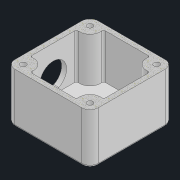
# Autodesk Inventor part: box
Saved by Autodesk Inventor 2021 (Build 250183000, 183)
## iProperties
Created: 2021-04-30
Part Number: box
Material: 一般
Document SubType Name: Modeling
Designer: yuta0
Density: 1 g/cm^3
Appearance: 既定
Author: yuta0
Autodesk Inventor part; units mm, degrees
ref_plane "YZ Plane" through (0, 0, 0) normal (1, 0, 0) x (0, 1, 0)
ref_plane "XZ Plane" through (0, 0, 0) normal (0, 1, 0) x (-1, 0, 0)
ref_plane "XY Plane" through (0, 0, 0) normal (0, 0, 1) x (1, 0, 0)
sketch "スケッチ1" plane through (0, 0, 0) normal (0, 1, 0) x (-1, 0, 0)
  line L0 (25, 25) -> (-25, 25)
  line L1 (-25, 25) -> (-25, -25)
  line L2 (-25, -25) -> (25, -25)
  line L3 (25, -25) -> (25, 25)
  line L4 (25, 25) -> (-25, -25) construction
  line L5 (-25, 25) -> (25, -25) construction
  point P0 (0, 0)
  dimension "d0" = 50
  dimension "d1" = 50
  constraints: 12 end point, 2 midpoint, 2 parallel, 1 horizontal, 1 perpendicular
  measures "d0" distance of L2.end L1.end
  measures "d1" distance of L1.end L0.end
extrude "押し出し1" add sketch "スケッチ1" against normal mid plane 33
fillet "フィレット1" radius 5 4 edges at (25, 0, 25) (25, 0, -25) (-25, 0, 25) (-25, 0, -25)
fillet "フィレット2" radius 1 16 edges at (25, -16.5, 0) (23.5355, -16.5, 23.5355) (0, -16.5, 25) (-23.5355, -16.5, 23.5355) (-25, -16.5, 0) (-23.5355, -16.5, -23.5355) (0, -16.5, -25) (23.5355, -16.5, -23.5355) (23.5355, 16.5, 23.5355) (25, 16.5, 0) (23.5355, 16.5, -23.5355) (0, 16.5, -25) (-23.5355, 16.5, -23.5355) (-25, 16.5, 0) (-23.5355, 16.5, 23.5355) (0, 16.5, 25)
sketch "スケッチ2" plane through (0, 16.5, 0) normal (0, 1, 0) x (1, 0, 0)
  arc A0 (-25, -20) -> (-20, -25) centre (-20, -20) ccw projected
  arc A1 (-20, 25) -> (-25, 20) centre (-20, 20) ccw projected
  arc A2 (25, 20) -> (20, 25) centre (20, 20) ccw projected
  arc A3 (20, -25) -> (25, -20) centre (20, -20) ccw projected
  point P0 (0, 0)
hole "穴1" at (-20, 16.5, -20) at (20, 16.5, 20) at (-20, 16.5, 20) at (20, 16.5, -20) direction (0, -1, 0) diameter 3.4 end through all counterbore diameter 6.5 counterbore depth 3 clearance for "Socket Head Cap Screw" size "M3" standard "Ansi Metric M Profile"
shell "シェル1" thickness 3 removed faces 0
sketch "スケッチ3" plane through (0, -16.5, 0) normal (0, -1, 0) x (1, 0, 0)
  circle A0 centre (20, 20) radius 1.7 projected
  circle A1 centre (-20, 20) radius 1.7 projected
  circle A2 centre (-20, -20) radius 1.7 projected
  line L0 (21.5877, 17.25) -> (18.4123, 17.25)
  line L1 (18.4123, 17.25) -> (16.8246, 20)
  line L2 (16.8246, 20) -> (18.4123, 22.75)
  line L3 (18.4123, 22.75) -> (21.5877, 22.75)
  line L4 (21.5877, 22.75) -> (23.1754, 20)
  line L5 (23.1754, 20) -> (21.5877, 17.25)
  line L6 (-20, 24) -> (20, 24) projected
  circle A3 centre (20, -20) radius 1.7 projected
  line L7 (21.5877, -17.25) -> (23.1754, -20)
  line L8 (23.1754, -20) -> (21.5877, -22.75)
  line L9 (21.5877, -22.75) -> (18.4123, -22.75)
  line L10 (18.4123, -22.75) -> (16.8246, -20)
  line L11 (16.8246, -20) -> (18.4123, -17.25)
  line L12 (18.4123, -17.25) -> (21.5877, -17.25)
  line L13 (-18.4123, -22.75) -> (-21.5877, -22.75)
  line L14 (-21.5877, -22.75) -> (-23.1754, -20)
  line L15 (-23.1754, -20) -> (-21.5877, -17.25)
  line L16 (-21.5877, -17.25) -> (-18.4123, -17.25)
  line L17 (-18.4123, -17.25) -> (-16.8246, -20)
  line L18 (-16.8246, -20) -> (-18.4123, -22.75)
  line L19 (-21.5877, 22.75) -> (-18.4123, 22.75)
  line L20 (-18.4123, 22.75) -> (-16.8246, 20)
  line L21 (-16.8246, 20) -> (-18.4123, 17.25)
  line L22 (-18.4123, 17.25) -> (-21.5877, 17.25)
  line L23 (-21.5877, 17.25) -> (-23.1754, 20)
  line L24 (-23.1754, 20) -> (-21.5877, 22.75)
  point P0 (0, 0)
  dimension "d14" = 5.5
  dimension "d15" = 5.5
  dimension "d16" = 5.5
  dimension "d17" = 5.5
  constraints: 48 end point, 4 coincident, 4 parallel, 52 other
  measures "d14" distance between parallel lines of L3 L0
  measures "d15" distance between parallel lines of L22 L19
  measures "d16" distance between parallel lines of L13 L16
  measures "d17" distance between parallel lines of L9 L12
extrude "押し出し2" cut sketch "スケッチ3" against normal blind 3 contours A0 | A1 | A2 | L0 L1 L2 L3 L4 L5 | A3 | L7 L8 L9 L10 L11 L12 | L13 L14 L15 L16 L17 L18 | L19 L20 L21 L22 L23 L24
sketch "スケッチ4" plane through (0, 16.5, 0) normal (0, 1, 0) x (1, 0, 0)
  circle A0 centre (0, 0) radius 8.1
  circle A1 centre (-7.8, 0) radius 1.6
  circle A2 centre (0, -7.8) radius 1.6
  circle A3 centre (7.8, 0) radius 1.6
  circle A4 centre (0, 7.8) radius 1.6
  point P0 (-7.9417, -1.5937)
  point P1 (-7.9417, 1.5937)
  point P2 (-1.5937, 7.9417)
  point P3 (1.5937, 7.9417)
  point P4 (7.9417, -1.5937)
  point P5 (7.9417, 1.5937)
  point P6 (1.5937, -7.9417)
  point P7 (-1.5937, -7.9417)
  dimension "d20" = 16.2
  dimension "d30" = 7.8
  dimension "d31" = 3.2
  dimension "d35" = 360
  constraints: 5 centre point, 1 coincident, 1 horizontal alignment, 9 other
  measures "d20" diameter of A0
  measures "d30" distance of A0.centre A1.centre
  measures "d31" diameter of A1
extrude "押し出し3" cut sketch "スケッチ4" against normal blind 3
sketch "スケッチ6" plane through (-25, -15.5, -20) normal (-1, 0, 0) x (0, 0, 1)
  circle A0 centre (20, 11.5) radius 8
  line L0 (0, -1) -> (40, -1) projected
  circle A1 centre (20, 11.5) radius 9.5 construction
  line L1 (16.7274, 4.2) -> (23.2726, 4.2)
  point P0 (20, 15.5)
  dimension "d26" = 16
  dimension "d27" = 12.5
  dimension "d37" = 19
  dimension "d38" = 7.3
  constraints: 2 centre point, 2 end point, 2 point on circle, 1 coincident, 1 horizontal, 1 vertical alignment
  measures "d26" diameter of A0
  measures "d27" distance from line of L0 A0.centre
  measures "d37" diameter of A1
  measures "d38" distance from line of A0.centre L1
extrude "押し出し5" cut sketch "スケッチ6" against normal blind 3 contours A0 L1 picked at (19.7393, 9.2872)
fillet "フィレット4" radius 1 8 edges at (-7.9417, 15, 1.5937) (-7.9417, 15, -1.5937) (-1.5937, 15, -7.9417) (1.5937, 15, -7.9417) (7.9417, 15, -1.5937) (7.9417, 15, 1.5937) (1.5937, 15, 7.9417) (-1.5937, 15, 7.9417)
sketch "スケッチ7" plane through (-15.7468, -13.5, -22) normal (0, 1, 0) x (1, 0, 0)
  arc A0 (1.6681, -44) -> (-6.2532, -36.0786) centre (-4.2532, -42) ccw projected
  line L0 (-6.2532, -18.7274) -> (-6.2532, -25.2726) projected
  line L1 (-6.2532, -25.2726) -> (-6.2532, -18.7274) projected
  line L2 (-6.2532, -6.2532) -> (-6.2532, -7.9214) projected
  line L3 (-6.2532, -7.9214) -> (-6.2532, -36.0786) projected
  line L4 (-6.2532, -36.0786) -> (-6.2532, -37.7468) projected
  line L5 (-6.2532, -37.7468) -> (-6.2532, -6.2532) projected
  arc A1 (-6.2532, -7.9214) -> (1.6681, 0) centre (-4.2532, -2) ccw projected
  line L6 (31.4935, 0) -> (29.8254, 0) projected
  line L7 (29.8254, 0) -> (1.6681, 0) projected
  line L8 (1.6681, 0) -> (0, 0) projected
  line L9 (0, 0) -> (31.4935, 0) projected
  arc A2 (29.8254, 0) -> (37.7468, -7.9214) centre (35.7468, -2) ccw projected
  arc A3 (37.7468, -36.0786) -> (29.8254, -44) centre (35.7468, -42) ccw projected
  line L10 (31.4935, -44) -> (0, -44) projected
  line L11 (0, -44) -> (1.6681, -44) projected
  line L12 (1.6681, -44) -> (29.8254, -44) projected
  line L13 (29.8254, -44) -> (31.4935, -44) projected
  line L14 (37.7468, -37.7468) -> (37.7468, -6.2532) projected
  line L15 (37.7468, -37.7468) -> (37.7468, -36.0786) projected
  line L16 (37.7468, -36.0786) -> (37.7468, -7.9214) projected
  line L17 (37.7468, -7.9214) -> (37.7468, -6.2532) projected
  arc A4 (0, -44) -> (-6.2532, -37.7468) centre (-4.2532, -42) ccw projected
  arc A5 (-6.2532, -6.2532) -> (0, 0) centre (-4.2532, -2) ccw projected
  arc A6 (31.4935, 0) -> (37.7468, -6.2532) centre (35.7468, -2) ccw projected
  arc A7 (37.7468, -37.7468) -> (31.4935, -44) centre (35.7468, -42) ccw projected
  point P0 (15.7468, -22)
  point P1 (1.6681, -44)
  point P2 (37.7468, -36.0786)
extrude "押し出し6" add sketch "スケッチ7" along normal up to surface (24 mm away) contours L10 A4 L4 A0 | A3 L14 A7 L10 | A2 L6 A6 L14 | L2 A5 L8 A1
fillet "フィレット5" radius 1 24 edges at (-22, 12, 14.0786) (-22, 3.0124, 14.0786) (-22, -8.9876, 14.0786) (-14.0786, 12, 22) (-14.0786, -8.9876, 22) (-14.0786, 3.0124, 22) (-22, -8.9876, -14.0786) (-22, 3.0124, -14.0786) (-22, 12, -14.0786) (-14.0786, 12, -22) (-14.0786, 3.0124, -22) (-14.0786, -8.9876, -22) (14.0786, -8.9876, -22) (14.0786, 3.0124, -22) (14.0786, 12, -22) (22, 12, -14.0786) (22, 3.0124, -14.0786) (22, -8.9876, -14.0786) (22, 12, 14.0786) (22, -8.9876, 14.0786) (22, 3.0124, 14.0786) (14.0786, 12, 22) (14.0786, 3.0124, 22) (14.0786, -8.9876, 22)
equation "\"d15\" = d14"
equation "\"d16\" = d14"
equation "\"d17\" = d14"
